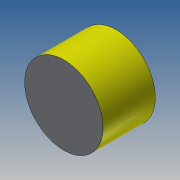
# Autodesk Inventor part: Honeypot
Saved by Autodesk Inventor 2015 (Build 190159000, 159)
## iProperties
Created: 2014-12-14
Part Number: Honeypot
Material: Generic
Document SubType Name: Modeling
Designer: Flopy
Density: 1 g/cm^3
Appearance: Default
Author: Flopy
Autodesk Inventor part; units mm, degrees
ref_plane "YZ Plane" through (0, 0, 0) normal (1, 0, 0) x (0, 1, 0)
ref_plane "XZ Plane" through (0, 0, 0) normal (0, 1, 0) x (-1, 0, 0)
ref_plane "XY Plane" through (0, 0, 0) normal (0, 0, 1) x (1, 0, 0)
sketch "Sketch1" plane through (0, 0, 0) normal (0, 0, 1) x (1, 0, 0)
  line L0 (0, 0) -> (150, 0)
  line L1 (150, 0) -> (150, 200)
  line L2 (150, 200) -> (145, 200)
  line L3 (145, 200) -> (145, 180)
  line L4 (145, 180) -> (0, 180)
  line L5 (0, 180) -> (0, 0)
  dimension "d0" = 300
  dimension "d1" = 200
  dimension "d2" = 5
  dimension "d3" = 20
  constraints: 12 end point, 4 perpendicular, 1 horizontal, 1 vertical
  measures "d0" diameter of L1 L5
  measures "d1" distance of L0.end L1.end
  measures "d2" distance of L1.end L2.end
  measures "d3" distance from line of L1.end L4
revolve "Revolution1" add sketch "Sketch1" angle 360 about axis through (0, 180, 0) along (0, -1, 0)
body "Solid1"
